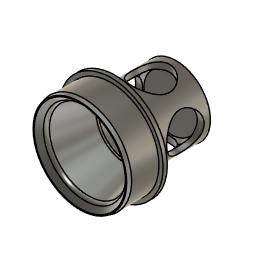
Abschlussstopfen v2 (Autodesk Fusion 360 design; units mm, degrees)
Autodesk Fusion 360 part; units mm, degrees
sketch "Skizze1" plane through (0, 0, 0) normal (0, 0, 1) x (1, 0, 0)
  line L0 (-23, 1.866) -> (-23, 15)
  line L1 (-23, 15) -> (-25, 15)
  line L2 (-25, 15) -> (-25, 17)
  line L3 (0, 59.1339) -> (0, 0) construction
  line L4 (-22, 0) -> (-22.5, 0)
  line L5 (-22, 0) -> (-19, 3)
  line L6 (-19, 3) -> (-13.9924, 22.363)
  line L7 (-13.9924, 22.363) -> (-13.9924, 43.7514)
  line L8 (-13.9924, 43.7514) -> (-1.5, 43.7514)
  line L9 (-25, 17) -> (-20.5, 17)
  line L10 (-20.5, 17) -> (-20.5, 7.1848)
  line L11 (-20.5, 7.1848) -> (-16.4924, 22.681)
  line L12 (-16.4924, 22.681) -> (-16.4924, 46.2514)
  line L13 (-16.4924, 46.2514) -> (-1.5, 46.2514)
  line L14 (-1.5, 43.7514) -> (-1.5, 46.2514)
  line L15 (0, 0) -> (-22.5, 0) construction
  line L16 (-22.5, 0) -> (-23, 1.866)
  dimension "d1" = 23
  dimension "d3" = 2
  dimension "d4" = 2
  dimension "d10" = 45
  dimension "d14" = 14.5
  dimension "d15" = 20
  dimension "d16" = 19
  dimension "d17" = 2.5
  dimension "d19" = 2.5
  dimension "d20" = 2.5
  dimension "d21" = 2.5
  dimension "d22" = 1.5
  dimension "d23" = 15
  constraint vertical L0
  constraint perpendicular L0 L1
  constraint perpendicular L1 L2
  constraint coincident L3.end L15.start
  constraint perpendicular L0 L4
  constraint vertical L7
  constraint perpendicular L2 L9
  constraint perpendicular L9 L10
  constraint parallel L7 L12
  constraint parallel L6 L11
  constraint perpendicular L12 L13
  constraint perpendicular L13 L14
  constraint perpendicular L3 L15
  measures "d1" distance of L0 L3
  measures "d3" distance of L0.end L1.end
  measures "d4" distance of L1.end L2.end
  measures "d10" angle of L4 L5
  measures "d14" angle of L3 L6
  measures "d15" distance of L5.end L6.end
  measures "d16" distance of L3 L5.end
  measures "d17" distance of L0 L10
  measures "d19" distance of L6 L11
  measures "d20" distance of L7 L12
  measures "d21" distance of L8 L13
  measures "d22" distance of L3 L14
  measures "d23" angle of L0 L16
revolve "Drehen1" add sketch "Skizze1" angle 360 about axis through (0, 59.1339, 0) along (0, -1, 0)
fillet "Abrundung1" radius 4 1 edges at (-17.7142, 3, 6.8707)
chamfer "Fase1" distance 1 angle 45 1 edges at (-1.3985, 43.7514, 0.5424)
fillet "Abrundung2" radius 4 1 edges at (-13.0455, 22.363, 5.0599)
chamfer "Fase2" distance 3 distance2 1 1 edges at (-13.0455, 43.7514, 5.0599) measured on face at (-13.019, 36.7915, 5.1277)
sketch "Skizze2" plane through (0, 0, 0) normal (0, 0, 1) x (1, 0, 0)
  line L0 (0, 57.0662) -> (0, -9.8119) construction
  circle A0 centre (0, 34.148) radius 9
  line L1 (16.4924, 46.2514) -> (-16.4924, 46.2514)
  line L2 (18.4666, 43.148) -> (-20, 43.148) construction
  dimension "d33" = 18
  constraint vertical L0
  constraint coincident origin L0
  constraint coincident L0 A0.centre
  constraint horizontal L2
  constraint tangent A0 L2
  measures "d33" diameter of A0
extrude "Extrusion1" cut sketch "Skizze2" against normal blind 55 from surface at 20
sketch "Skizze3" plane through (0, 0, 0) normal (1, 0, 0) x (0, 1, 0)
  line L0 (52.8501, 0) -> (-11.2944, 0) construction
  line L1 (46.2514, -16.4924) -> (46.2514, 16.4924)
  line L2 (46.2514, -1.5) -> (46.2514, 1.5)
  circle A0 centre (34.2514, 0) radius 9
  line L3 (43.2514, 22) -> (43.2514, -22.5181) construction
  dimension "d37" = 18
  dimension "d38" = 3
  constraint horizontal L0
  constraint coincident origin L0
  constraint coincident L0 A0.centre
  constraint parallel L1 L3
  constraint tangent A0 L3
  measures "d37" diameter of A0
  measures "d38" distance of L1 L3
extrude "Extrusion2" cut sketch "Skizze3" along normal blind 65 from surface at -30
equation "d1 = ( 46 / 2 ) * 1 mm"
equation "d16 = ( 38 / 2 ) * 1 mm"
